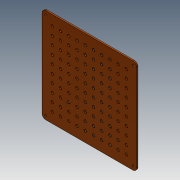
# Autodesk Inventor part: VP RAM NUT CAPTURE PLATE
Saved by Autodesk Inventor 2018.3 (Build 223284000, 284)
## iProperties
Created: 2018-09-09
Material: Generic
Vendor: HHMI: JRC - ID&F
Document SubType Name: Modeling
Designer: arnoldj
Density: 1 g/cm^3
Appearance: Smooth - Light Orange
RuleStatus: InUse
AfterDocSave0: file://Part Number Cleaner
DESIGN DEPARTMENT: HHMI: JRC - ID&F
ALTERED ITEM PART NUMBER: N/A
ALTERED ITEM VENDOR: N/A
ALTERED ITEM DESCRIPTION: N/A
Author: arnoldj
Revision Number: 0
Autodesk Inventor part; units mm, degrees
ref_plane "YZ Plane" through (0, 0, 0) normal (1, 0, 0) x (0, 1, 0)
ref_plane "XZ Plane" through (0, 0, 0) normal (0, 1, 0) x (-1, 0, 0)
ref_plane "XY Plane" through (0, 0, 0) normal (0, 0, 1) x (1, 0, 0)
sketch "Sketch1" plane through (0, 0, 0) normal (0, 0, 1) x (1, 0, 0)
  line L0 (0, 231.14) -> (0, -231.14) projected
  line L1 (-231.14, 0) -> (231.14, 0) projected
  line L2 (165.1, -165.1) -> (-165.1, -165.1)
  line L3 (-165.1, -165.1) -> (-165.1, 165.1)
  line L4 (-165.1, 165.1) -> (165.1, 165.1)
  line L5 (165.1, 165.1) -> (165.1, -165.1)
  line L6 (165.1, -165.1) -> (-165.1, 165.1) construction
  line L7 (-165.1, -165.1) -> (165.1, 165.1) construction
  line L8 (129.159, -129.159) -> (-129.159, -129.159)
  line L9 (-129.159, -129.159) -> (-129.159, 129.159)
  line L10 (-129.159, 129.159) -> (129.159, 129.159)
  line L11 (129.159, 129.159) -> (129.159, -129.159)
  line L12 (129.159, -129.159) -> (-129.159, 129.159) construction
  line L13 (-129.159, -129.159) -> (129.159, 129.159) construction
  line L14 (76.2, -76.2) -> (-76.2, -76.2) construction
  line L15 (-76.2, -76.2) -> (-76.2, 76.2) construction
  line L16 (-76.2, 76.2) -> (76.2, 76.2) construction
  line L17 (76.2, 76.2) -> (76.2, -76.2) construction
  line L18 (76.2, -76.2) -> (-76.2, 76.2) construction
  line L19 (-76.2, -76.2) -> (76.2, 76.2) construction
  line L20 (114.808, -114.808) -> (-114.808, -114.808) construction
  line L21 (-114.808, -114.808) -> (-114.808, 114.808) construction
  line L22 (-114.808, 114.808) -> (114.808, 114.808) construction
  line L23 (114.808, 114.808) -> (114.808, -114.808) construction
  line L24 (114.808, -114.808) -> (-114.808, 114.808) construction
  line L25 (-114.808, -114.808) -> (114.808, 114.808) construction
  line L26 (152.4, -152.4) -> (-152.4, -152.4) construction
  line L27 (-152.4, -152.4) -> (-152.4, 152.4) construction
  line L28 (-152.4, 152.4) -> (152.4, 152.4) construction
  line L29 (152.4, 152.4) -> (152.4, -152.4) construction
  line L30 (-152.4, -152.4) -> (152.4, 152.4) construction
  line L31 (150.1998, -145.6199) -> (159.1801, -154.6002)
  line L32 (159.1801, -154.6002) -> (154.6002, -159.1801)
  line L33 (154.6002, -159.1801) -> (145.6199, -150.1998)
  line L34 (145.6199, -150.1998) -> (150.1998, -145.6199)
  line L35 (150.1998, -145.6199) -> (154.6002, -159.1801) construction
  line L36 (159.1801, -154.6002) -> (145.6199, -150.1998) construction
  circle A0 centre (-129.159, 129.159) radius 16.383 construction
  line L37 (-140.7435, 117.5745) -> (-117.5745, 140.7435) construction
  circle A1 centre (-129.159, 100.457) radius 16.383 construction
  line L38 (-143.3471, 108.6485) -> (-114.9709, 92.2655) construction
  line L39 (-133.4643, 131.6447) -> (-129.159, 134.1303)
  line L40 (-129.159, 134.1303) -> (-124.8537, 131.6447)
  line L41 (-124.8537, 131.6447) -> (-124.8537, 126.6733)
  line L42 (-124.8537, 126.6733) -> (-129.159, 124.1877)
  line L43 (-129.159, 124.1877) -> (-133.4643, 126.6733)
  line L44 (-133.4643, 126.6733) -> (-133.4643, 131.6447)
  line L45 (0, 0) -> (-165.1, 165.1) construction
  dimension "d0" = 129.159
  dimension "d1" = 129.159
  dimension "d2" = 330.2
  dimension "d23" = 152.4
  dimension "d36" = 114.808
  dimension "d63" = 304.8
  dimension "d64" = 6.477
  dimension "d65" = 12.7
  dimension "d97" = 32.766
  dimension "d98" = 45
  dimension "d99" = 30
  dimension "d100" = 28.702
  dimension "d122" = 8.6106
  constraints: 88 end point, 13 midpoint, 12 parallel, 11 coincident, 7 perpendicular, 5 horizontal, 4 point on circle, 4 point on line, 2 centre point, 1 equal radius, 1 vertical, 13 other
  measures "d0" distance from line of L0 L9.end
  measures "d1" distance from line of L1 L9.end
  measures "d2" distance of L3.end L4.end
  measures "d23" distance of L15.end L16.end
  measures "d36" distance from line of L0 L21.end
  measures "d63" distance of L27.end L28.end
  measures "d64" distance of L31.end L32.end
  measures "d65" distance of L31.start L31.end
  measures "d97" diameter of A0
  measures "d98" angle of L10 L37
  measures "d99" angle of L10 L38
  measures "d100" distance of A1.centre A0.centre
  measures "d122" distance between parallel lines of L41 L44
extrude "Extrusion1" add sketch "Sketch1" against normal blind 4.572 contours L4 L5 L1 L11 L10 L0 | L0 L10 L41 L40 L39 L44 L43 L9 L1 L3 L4 | L10 L11 L1 L0 | L0 L1 L9 L42 L41 L10 | L1 L11 L8 L0 | L0 L8 L9 L1 | L41 L42 L9 L10 | L10 L9 L43 L44 L39 L40 L41 | L1 L9 L8 L0 L2 L3 | L5 L2 L0 L8 L11 L1 | L31 L32 L33 L34
fillet "Fillet2" radius 12.7 4 edges at (-165.1, -165.1, -2.286) (165.1, -165.1, -2.286) (165.1, 165.1, -2.286) (-165.1, 165.1, -2.286)
hole "Hole6" at (-152.4, 152.4, 0) at (-152.4, -152.4, 0) at (152.4, -152.4, 0) at (152.4, 152.4, 0) direction (0, 0, -1) diameter 6.35 end through all
sketch "Sketch4" plane through (0, 0, -4.572) normal (0, 0, -1) x (-1, 0, 0)
  point P0 (0, 0)
  point P1 (76.2, 76.2)
  point P2 (76.2, -76.2)
  point P3 (-76.2, -76.2)
  point P4 (-76.2, 76.2)
hole "Hole10" at (-76.2, -76.2, -4.572) at (76.2, -76.2, -4.572) at (76.2, 76.2, -4.572) at (-76.2, 76.2, -4.572) direction (0, 0, 1) diameter 4.699 end through all
extrude "Extrusion4" cut sketch "Sketch1" against normal up to next contours L41 L42 L9 L10 | L10 L9 L43 L44 L39 L40 L41
pattern_linear "Rectangular Pattern3" count 10 spacing 28.702 along (1, 0, 0) count 10 spacing 28.702 along (0, -1, 0) of "Extrusion4"
equation "\"d1\" = d0"
body "Solid1"
